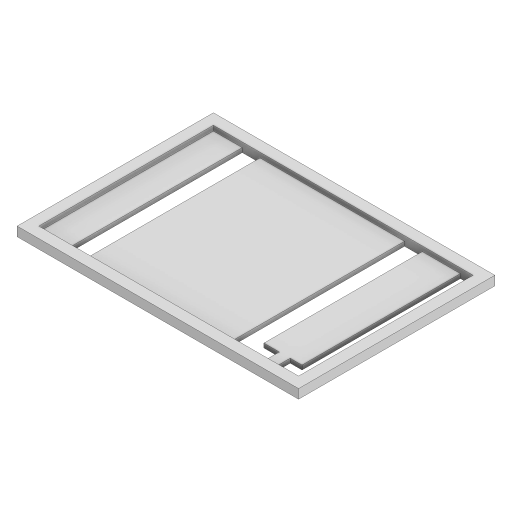
# Autodesk Inventor part: RFID_Bottom
Saved by Autodesk Inventor 2023 (Build 270158000, 158)
## iProperties
Created: 2022-10-13
Part Number: RFID_Bottom
Material: Generic
Document SubType Name: Modeling
Designer: Vking
Density: 1 g/cm^3
Appearance: Default
Author: Vking
Autodesk Inventor part; units mm, degrees
ref_plane "YZ Plane" through (0, 0, 0) normal (1, 0, 0) x (0, 1, 0)
ref_plane "XZ Plane" through (0, 0, 0) normal (0, 1, 0) x (-1, 0, 0)
ref_plane "XY Plane" through (0, 0, 0) normal (0, 0, 1) x (1, 0, 0)
sketch "Sketch1" plane through (0, 0, 0) normal (0, 1, 0) x (-1, 0, 0)
  line L0 (31, 20.5) -> (-30, 20.5)
  line L1 (-30, 20.5) -> (-30, -20.5)
  line L2 (-30, -20.5) -> (31, -20.5)
  line L3 (31, -20.5) -> (31, 20.5)
  line L4 (33.54, 23.04) -> (-32.54, 23.04)
  line L5 (-32.54, 23.04) -> (-32.54, -23.04)
  line L6 (-32.54, -23.04) -> (33.54, -23.04)
  line L7 (33.54, -23.04) -> (33.54, 23.04)
  line L8 (-12, -20.5) -> (-12, 20.5)
  line L9 (-12, -23.04) -> (-12, -20.5)
  line L10 (-12, 20.5) -> (-12, 23.04)
  point P0 (0, 0)
  dimension "d0" = 41
  dimension "d1" = 61
  dimension "d2" = 20.5
  dimension "d3" = 31
  dimension "d4" = 2.54
  dimension "d9" = 18
  constraints: 22 end point, 5 point on line, 4 parallel, 3 perpendicular, 1 horizontal, 1 vertical, 3 other
  measures "d0" distance of L2.end L0.start
  measures "d1" distance of L1.end L2.end
  measures "d2" distance from line of point (0, 0) L2
  measures "d3" distance from line of point (0, 0) L3
  measures "d4" distance between parallel lines of L3 L7
  measures "d9" distance between parallel lines of L1 L8
extrude "Extrusion1" add sketch "Sketch1" along normal blind 3.5 contours L0 L10 L4 L7 L6 L9 L2 L3
extrude "Extrusion3" add sketch "Sketch1" along normal blind 7 contours L0 L1 L2 L9 L6 L5 L4 L10
sketch "Sketch3" plane through (0, 0, 0) normal (0, -1, 0) x (1, 0, 0)
  line L0 (-31, -20.5) -> (30, -20.5) projected
  line L1 (-31, 20.5) -> (-31, -20.5) projected
  line L2 (30, 20.5) -> (-31, 20.5) projected
  line L3 (30, -20.5) -> (30, 20.5) projected
  line L4 (32.54, -23.04) -> (-33.54, -23.04) projected
  line L5 (32.54, 23.04) -> (32.54, -23.04) projected
  line L6 (-33.54, 23.04) -> (32.54, 23.04) projected
  line L7 (-33.54, -23.04) -> (-33.54, 23.04) projected
  point P0 (0, 0)
extrude "Extrusion4" add sketch "Sketch3" along normal blind 1 contours L1 L2 L3 L0 | L4 L7 L6 L5
sketch "Sketch4" plane through (0, 0, 0) normal (0, 1, 0) x (1, 0, 0)
  line L0 (12, -20.5) -> (-31, -20.5) projected
  line L1 (-31, -20.5) -> (-31, 20.5) projected
  line L2 (30, 20.5) -> (30, -20.5) projected
  line L3 (30, -20.5) -> (12, -20.5) projected
  line L4 (-31, 20.5) -> (12, 20.5) projected
  line L5 (-24.229, 20.5) -> (-20.038, 20.5)
  line L6 (-20.038, 20.5) -> (-20.038, -20.5)
  line L7 (-20.038, -20.5) -> (-24.229, -20.5)
  line L8 (-24.229, -20.5) -> (-24.229, 20.5)
  line L9 (18.062, -20.5) -> (13.871, -20.5)
  line L10 (13.871, -20.5) -> (13.871, 20.5)
  line L11 (13.871, 20.5) -> (18.062, 20.5)
  line L12 (18.062, 20.5) -> (18.062, -20.5)
  point P0 (0, 0)
  point P1 (11.52, -20.5)
  point P2 (-24.229, -20.5)
  point P3 (-20.038, 20.5)
  dimension "d30" = 33.909
  dimension "d31" = 4.191
  dimension "d37" = 4.191
  dimension "d38" = 11.938
  constraints: 16 end point, 4 parallel, 4 point on line, 2 horizontal, 2 perpendicular
  measures "d30" distance between parallel lines of L10 L6
  measures "d31" distance between parallel lines of L10 L12
  measures "d37" distance between parallel lines of L8 L6
  measures "d38" distance between parallel lines of L2 L12
extrude "Extrusion5" cut sketch "Sketch4" against normal blind 25.4 contours L0 L8 L4 L6 | L3 L10 L11 L12
sketch "Sketch5" plane through (-33.54, 3.5, 23.04) normal (0, 0, 1) x (1, 0, 0)
  line L0 (66.08, -4.5) -> (66.08, 3.5) projected
  line L1 (66.08, -2.3359) -> (-3.3215, -2.3359)
  line L2 (-3.3215, -2.3359) -> (-3.3215, 8.0283)
  line L3 (-3.3215, 8.0283) -> (66.08, 8.0283)
  line L4 (66.08, 8.0283) -> (66.08, -2.3359)
  point P0 (33.54, -3.5)
  point P1 (66.08, 3.5)
  constraints: 8 end point, 2 parallel, 1 horizontal, 1 perpendicular, 1 point on line
extrude "Extrusion6" cut sketch "Sketch5" against normal blind 76.2
sketch "Sketch6" plane through (0, 0, 0) normal (0, 1, 0) x (1, 0, 0)
  line L0 (30, 20.5) -> (-31, 20.5) projected
  line L1 (30, -20.5) -> (18.062, -20.5) projected
  line L2 (30, 20.5) -> (27, 20.5)
  line L3 (27, 20.5) -> (27, -20.5)
  line L4 (27, -20.5) -> (30, -20.5)
  line L5 (30, -20.5) -> (30, 20.5)
  point P0 (0, 0)
  dimension "d33" = 3
  constraints: 8 end point, 2 parallel, 1 horizontal, 1 perpendicular, 1 point on line
  measures "d33" distance between parallel lines of L5 L3
extrude "Extrusion7" cut sketch "Sketch6" against normal blind 25.4
sketch "Sketch7" plane through (0, 0, 0) normal (0, 1, 0) x (1, 0, 0)
  line L0 (13.871, -20.5) -> (18.062, -20.5) projected
  line L1 (27, -20.5) -> (27, 20.5) projected
  line L2 (18.062, -20.5) -> (27, -20.5)
  line L3 (27, -20.5) -> (27, -16.69)
  line L4 (27, -16.69) -> (18.062, -16.69)
  line L5 (18.062, -16.69) -> (18.062, -20.5)
  line L6 (27, -20.5) -> (18.062, -20.5) projected
  line L7 (21.6815, -16.69) -> (24.2215, -16.69)
  line L8 (24.2215, -16.69) -> (24.2215, -20.5)
  line L9 (24.2215, -20.5) -> (21.6815, -20.5)
  line L10 (21.6815, -20.5) -> (21.6815, -16.69)
  point P0 (0, 0)
  point P1 (21.6815, -20.5)
  dimension "d39" = 3.81
  dimension "d40" = 2.54
  dimension "d41" = 8.938
  dimension "d42" = 3.6195
  constraints: 16 end point, 4 parallel, 3 point on line, 2 horizontal, 2 perpendicular
  measures "d39" distance between parallel lines of L2 L4
  measures "d40" distance between parallel lines of L8 L10
  measures "d41" distance of L3.end L4.end
  measures "d42" distance between parallel lines of L10 L5
extrude "Extrusion8" cut sketch "Sketch7" against normal blind 25.4 contours L2 L8 L4 L1 | L2 L5 L4 L10
body "Solid1"
